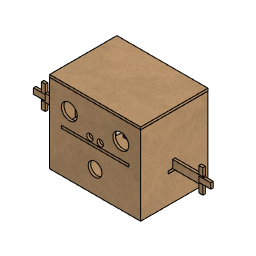
CAD finished (Autodesk Fusion 360 design; units mm, degrees)
Autodesk Fusion 360 part; units mm, degrees
sketch "Sketch1" plane through (0, 0, 0) normal (0, 0, 1) x (1, 0, 0)
  line L0 (-32.379468, 47.484339) -> (40, 47.484339)
  line L1 (40, 47.484339) -> (40, -5)
  line L2 (40, -5) -> (-32.379468, -5)
  line L3 (-32.379468, -5) -> (-32.379468, 47.484339)
  constraint horizontal L0
  constraint vertical L1
  constraint horizontal L2
  constraint vertical L3
sketch "Sketch2" plane through (0, 0, 0) normal (0, 0, 1) x (1, 0, 0)
sketch "Sketch3" plane through (0, 0, 0) normal (0, 0, 1) x (1, 0, 0)
  line L0 (-70, 30) -> (-16.7, 30)
  line L1 (-16.7, 30) -> (-16.7, -38.6)
  line L2 (-16.7, -38.6) -> (-70, -38.6)
  line L3 (-70, -38.6) -> (-70, 30)
  dimension "d3" = 53.3
  dimension "d4" = 68.6
  constraint horizontal L0
  constraint vertical L1
  constraint horizontal L2
  constraint vertical L3
  measures "d3" distance of L0.start L0.end
  measures "d4" distance of L0.start L2.end
extrude "Extrude2" add sketch "Sketch3" along normal blind 10 contours L0 L1 L2 L3 picked at (-34.466667, -15.733333) makes body 1
move_body "Move3" bodies 1 to x (0, -1, 0) y (1, 0, 0) z (0, 0, 1) at (-31.4, -108.6, 0)
move_body "Move4" bodies 1 to x (1, 0, 0) y (0, 1, 0) z (0, 0, 1) at (-5.934669, 58.827333, -1.64215)
sketch "Sketch4" plane through (0, 0, 0) normal (0, 0, 1) x (1, 0, 0)
  line L0 (40, 25) -> (125, 25)
  line L1 (125, 25) -> (125, -30)
  line L2 (125, -30) -> (40, -30)
  line L3 (40, -30) -> (40, 25)
  dimension "d7" = 85
  dimension "d8" = 55
  constraint horizontal L0
  constraint vertical L1
  constraint horizontal L2
  constraint vertical L3
  measures "d7" distance of L0.start L0.end
  measures "d8" distance of L0.start L2.end
extrude "Extrude3" add sketch "Sketch4" along normal blind 10 separate body contours L0 L1 L2 L3 picked at (68.333333, 6.666667) makes body 2
move_body "Move5" bodies 1 to x (0, 1, 0) y (-1, 0, 0) z (0, 0, 1) at (-109.007335, 42.862002, 0)
move_body "Move6" bodies 1 to x (1, 0, 0) y (0, 1, 0) z (0, 0, 1) at (69.290138, 3.072667, 11.64215)
move_body "Move7" bodies 2 to x (0, 1, 0) y (-1, 0, 0) z (0, 0, 1) at (10, -70, 0)
move_body "Move8" bodies 2 to x (1, 0, 0) y (0, 1, 0) z (0, 0, 1) at (13.481554, 0.965731, 8.735429)
sketch "Sketch5" plane through (0, 0, 0) normal (0, 0, 1) x (1, 0, 0)
  line L0 (100, -150) -> (-130, -150)
  line L1 (-130, -150) -> (-130, 20)
  line L2 (-130, 20) -> (100, 20)
  line L3 (100, 20) -> (100, -150)
  dimension "d11" = 230
  dimension "d12" = 170
  constraint horizontal L0
  constraint vertical L1
  constraint horizontal L2
  constraint vertical L3
  measures "d11" distance of L0.start L0.end
  measures "d12" distance of L0.start L2.end
extrude "Extrude4" add sketch "Sketch5" against normal blind 200 separate body contours L0 L1 L2 L3 picked at (-53.333333, -93.333333) makes body 3
sketch "Sketch6" plane through (0, 0, -200) normal (0, 0, -1) x (1, 0, 0)
  line L0 (-130, -20) -> (100, -20)
  line L1 (100, -20) -> (100, 150)
  line L2 (100, 150) -> (-130, 150)
  line L3 (-130, 150) -> (-130, -20)
  line L4 (-122.888911, 140.96297) -> (94.411089, 140.96297)
  line L5 (94.411089, 140.96297) -> (94.411089, -12.73703)
  line L6 (94.411089, -12.73703) -> (-122.888911, -12.73703)
  line L7 (-122.888911, -12.73703) -> (-122.888911, 140.96297)
  dimension "d15" = 217.3
  dimension "d16" = 153.7
  constraint horizontal L4
  constraint vertical L5
  constraint horizontal L6
  constraint vertical L7
extrude "Extrude5" cut sketch "Sketch6" against normal blind 193.35 contours L4 L5 L6 L7 picked at (-50.455578, 89.729637) bodies 3
move_body "Move9" bodies 1 to x (1, 0, 0) y (0, 1, 0) z (0, 0, 1) at (-192.155267, -38.643573, -133.723853)
move_body "Move10" bodies 2 to x (1, 0, 0) y (0, 1, 0) z (0, 0, 1) at (-190.142564, -42.930176, -139.080704)
sketch "Sketch7" plane through (0, 0, 0) normal (0, 0, 1) x (1, 0, 0)
  line L0 (-116.722098, 87.554715) -> (113.277902, 87.554715)
  line L1 (113.277902, 87.554715) -> (113.277902, 257.554715)
  line L2 (113.277902, 257.554715) -> (-116.722098, 257.554715)
  line L3 (-116.722098, 257.554715) -> (-116.722098, 87.554715)
  dimension "d19" = 230
  dimension "d20" = 170
  constraint horizontal L0
  constraint vertical L1
  constraint horizontal L2
  constraint vertical L3
extrude "Extrude6" add sketch "Sketch7" along normal blind 6.35 separate body contours L0 L1 L2 L3 picked at (-40.055431, 200.888048) makes body 4
move_body "Move11" bodies 4 to x (1, 0, 0) y (0, 1, 0) z (0, 0, 1) at (-13.20842, -237.892283, -206.176126)
sketch "Sketch8" plane through (0, 20, 0) normal (0, 1, 0) x (-1, 0, 0)
  line L0 (130, 0) -> (-100, 0)
  line L1 (-100, 0) -> (-100, -200)
  line L2 (-100, -200) -> (130, -200)
  line L3 (130, -200) -> (130, 0)
  line L4 (100, -110) -> (-72.739623, -110)
  line L5 (-72.739623, -110) -> (-72.739623, -103.65)
  line L6 (-72.739623, -103.65) -> (100, -103.65)
  line L7 (100, -103.65) -> (100, -110)
  dimension "d23" = 6.35
  constraint horizontal L4
  constraint vertical L5
  constraint horizontal L6
  constraint vertical L7
  measures "d23" distance of L4.start L6.end
extrude "Extrude7" cut sketch "Sketch8" against normal blind 200 contours L4 L5 L6 L7 picked at (42.420126, -107.883333) bodies 3
sketch "Sketch9" plane through (0, 0, 0) normal (0, 0, 1) x (1, 0, 0)
  line L0 (-120, 110) -> (52.74, 110)
  line L1 (52.74, 110) -> (52.74, 280)
  line L2 (52.74, 280) -> (-120, 280)
  line L3 (-120, 280) -> (-120, 110)
  dimension "d26" = 172.74
  dimension "d27" = 170
  constraint horizontal L0
  constraint vertical L1
  constraint horizontal L2
  constraint vertical L3
  measures "d26" distance of L0.start L0.end
  measures "d27" distance of L0.start L2.end
extrude "Extrude8" add sketch "Sketch9" against normal blind 6.35 separate body contours L0 L1 L2 L3 picked at (-62.42, 166.666667) makes body 5
move_body "Move12" bodies 5 to x (1, 0, 0) y (0, 1, 0) z (0, 0, 1) at (20.106965, -259.503239, -103.236774)
sketch "Sketch10" plane through (0, -150, 0) normal (0, -1, 0) x (1, 0, 0)
  line L0 (72.739623, -103.65) -> (72.739623, -110)
  line L1 (72.739623, -110) -> (-100, -110)
  line L2 (-100, -110) -> (-100, -103.65)
  line L3 (-100, -103.65) -> (72.739623, -103.65)
  line L4 (100, 0) -> (-130, 0)
  line L5 (-130, 0) -> (-130, -200)
  line L6 (-130, -200) -> (100, -200)
  line L7 (100, -200) -> (100, 0)
  circle A0 centre (50, -150) radius 20
  circle A1 centre (50, -150) radius 20
  circle A2 centre (-80, -150) radius 20
extrude "Extrude9" cut sketch "Sketch10" against normal blind 20 contours A0 A1 | A2 picked at (55.729979, -143.285883) picked at (-74.270021, -143.285883) bodies 3
sketch "Sketch11" plane through (0, -150, 0) normal (0, -1, 0) x (1, 0, 0)
  circle A0 centre (-80, -150) radius 20
  circle A1 centre (50, -150) radius 20
  line L0 (72.739623, -103.65) -> (72.739623, -110)
  line L1 (72.739623, -110) -> (-100, -110)
  line L2 (-100, -110) -> (-100, -103.65)
  line L3 (-100, -103.65) -> (72.739623, -103.65)
  line L4 (100, 0) -> (-130, 0)
  line L5 (-130, 0) -> (-130, -200)
  line L6 (-130, -200) -> (100, -200)
  line L7 (100, -200) -> (100, 0)
  circle A2 centre (-1.949729, -120.049809) radius 8.05
  dimension "d32" = 16.1
  measures "d32" diameter of A2
sketch "Sketch12" plane through (0, -150, 0) normal (0, -1, 0) x (1, 0, 0)
sketch "Sketch13" plane through (0, -150, 0) normal (0, -1, 0) x (1, 0, 0)
  circle A0 centre (-28.05, -120.05) radius 8.05
  dimension "d33" = 16.1
  measures "d33" diameter of A0
extrude "Extrude10" cut sketch "Sketch11" sketch "Sketch13" against normal blind 10 contours A2 picked at (-2.546826, -117.670176) of sketch 2 contours A0 picked at (-28.647098, -117.433943) bodies 3
move_body "Move13" bodies 4 to x (1, 0, 0) y (0, 1, 0) z (0, 0, 1) at (231.754055, -19.247754, 6.176126)
move_body "Move14" bodies 2 to x (1, 0, 0) y (0, 1, 0) z (0, 0, 1) at (189.899012, -32.028626, 10.567885)
move_body "Move15" bodies 1 to x (1, 0, 0) y (0, 1, 0) z (0, 0, 1) at (183.687801, -30.675834, -12.288573)
move_body "Move16" bodies 1 to x (1, 0, 0) y (0, 1, 0) z (0, 0, 1) at (0, 0, 15)
sketch "Sketch14" plane through (100, 0, 0) normal (1, 0, 0) x (0, 1, 0)
sketch "Sketch15" plane through (100, 0, 0) normal (1, 0, 0) x (0, 1, 0)
  line L0 (-50, -75) -> (-80, -75)
  line L1 (-80, -75) -> (-80, -68.65)
  line L2 (-80, -68.65) -> (-50, -68.65)
  line L3 (-50, -68.65) -> (-50, -75)
  dimension "d36" = 6.35
  constraint horizontal L0
  constraint vertical L1
  constraint horizontal L2
  constraint vertical L3
  measures "d36" distance of L0.start L2.end
extrude "Extrude11" cut sketch "Sketch15" against normal blind 320 contours L0 L1 L2 L3 picked at (-70, -72.883333) bodies 3
sketch "Sketch16" plane through (0, 0, 0) normal (0, 0, 1) x (1, 0, 0)
  line L0 (-100, 140) -> (130, 140)
  line L1 (130, 140) -> (130, 170)
  line L2 (130, 170) -> (-100, 170)
  line L3 (-100, 170) -> (-100, 140)
  dimension "d39" = 230
  dimension "d40" = 30
  constraint horizontal L0
  constraint vertical L1
  constraint horizontal L2
  constraint vertical L3
  measures "d39" distance of L0.start L0.end
  measures "d40" distance of L0.start L2.end
extrude "Extrude12" add sketch "Sketch16" against normal blind 6.35 separate body contours L0 L1 L2 L3 picked at (-23.333333, 150) makes body 6
move_body "Move17" bodies 6 to x (1, 0, 0) y (0, 1, 0) z (0, 0, 1) at (-29.739923, -217.865341, -68.375414)
move_body "Move18" bodies 6 to x (1, 0, 0) y (0, 1, 0) z (0, 0, 1) at (0, -2.152, 0)
sketch "Sketch17" plane through (0, 0, -74.725414) normal (0, 0, -1) x (1, 0, 0)
  line L0 (-129.739923, 80.017341) -> (-129.739923, 50.017341)
  line L1 (-129.739923, 50.017341) -> (100.260077, 50.017341)
  line L2 (100.260077, 50.017341) -> (100.260077, 80.017341)
  line L3 (100.260077, 80.017341) -> (-129.739923, 80.017341)
sketch "Sketch18" plane through (0, 0, -74.725414) normal (0, 0, -1) x (1, 0, 0)
  line L0 (90.260001, 76.717001) -> (86.610001, 76.717001)
  line L1 (86.610001, 76.717001) -> (86.610001, 64.717001)
  line L2 (86.610001, 64.717001) -> (90.260001, 64.717001)
  line L3 (90.260001, 64.717001) -> (90.260001, 76.717001)
  dimension "d43" = 3.65
  constraint horizontal L0
  constraint vertical L1
  constraint horizontal L2
  constraint vertical L3
sketch "Sketch19" plane through (0, 0, -74.725414) normal (0, 0, -1) x (1, 0, 0)
  line L0 (60.610001, 64.717001) -> (56.960001, 64.717001)
  line L1 (56.960001, 64.717001) -> (56.960001, 76.717001)
  line L2 (56.960001, 76.717001) -> (60.610001, 76.717001)
  line L3 (60.610001, 76.717001) -> (60.610001, 64.717001)
  dimension "d44" = 3.65
  constraint horizontal L0
  constraint vertical L1
  constraint horizontal L2
  constraint vertical L3
extrude "Extrude13" cut sketch "Sketch18" against normal blind 11 contours L0 L1 L2 L3 picked at (87.826668, 72.717001) bodies 6
extrude "Extrude14" cut sketch "Sketch19" against normal blind 22 contours L0 L1 L2 L3 picked at (58.176668, 68.717001) bodies 6
sketch "Sketch20" plane through (0, 0, 0) normal (0, 0, 1) x (1, 0, 0)
  line L0 (95, -105) -> (91.35, -105)
  line L1 (91.35, -105) -> (91.35, -117)
  line L2 (91.35, -117) -> (95, -117)
  line L3 (95, -117) -> (95, -105)
  dimension "d49" = 3.65
  dimension "d50" = 12
  constraint horizontal L0
  constraint vertical L1
  constraint horizontal L2
  constraint vertical L3
  measures "d49" distance of L0.start L0.end
  measures "d50" distance of L0.start L2.end
sketch "Sketch21" plane through (0, 0, 0) normal (0, 0, 1) x (1, 0, 0)
  line L0 (65.35, -105) -> (61.7, -105)
  line L1 (61.7, -105) -> (61.7, -117)
  line L2 (61.7, -117) -> (65.35, -117)
  line L3 (65.35, -117) -> (65.35, -105)
  dimension "d51" = 3.65
  dimension "d52" = 12
  constraint horizontal L0
  constraint vertical L1
  constraint horizontal L2
  constraint vertical L3
  measures "d51" distance of L0.start L0.end
  measures "d52" distance of L0.start L2.end
extrude "Extrude15" add sketch "Sketch21" against normal blind 25 separate body contours L0 L1 L2 L3 picked at (62.916667, -109) makes body 7
extrude "Extrude16" add sketch "Sketch20" against normal blind 25 separate body contours L0 L1 L2 L3 picked at (92.566667, -109) makes body 8
extrude "Extrude17" cut 1 faces at (86.610001, -72.717001, -72.608747) along direction (-1, 0, 0) blind 2.65 on bodies 6 bodies 6
extrude "Extrude18" cut 1 faces at (83.960001, -72.717001, -72.608747) along direction (-1, 0, 0) blind 0.05 on bodies 6 bodies 6
extrude "Extrude19" cut 1 faces at (56.960001, -68.717001, -72.608747) along direction (-1, 0, 0) blind 6.35 on bodies 6 bodies 6
extrude "Extrude20" add 1 faces at (60.610001, -72.717001, -72.608747) along direction (-1, 0, 0) blind 3.3 on bodies 6 bodies 6
extrude "Extrude21" cut 1 faces at (57.310001, -72.717001, -72.608747) along direction (1, 0, 0) blind 0.6 on bodies 6 bodies 6
extrude "Extrude22" add 1 faces at (50.610001, -68.717001, -72.608747) along direction (1, 0, 0) blind 0.95 on bodies 6 bodies 6
extrude "Extrude23" add 1 faces at (91.35, -109, -8.333333) along direction (-1, 0, 0) blind 0.7 on bodies 8 bodies 8
extrude "Extrude24" cut 1 faces at (65.35, -113, -8.333333) along direction (-1, 0, 0) blind 0.7 on bodies 7 bodies 7
extrude "Extrude25" add 1 faces at (61.7, -109, -8.333333) along direction (-1, 0, 0) blind 1.4 on bodies 7 bodies 7
extrude "Extrude26" add 1 faces at (90.65, -109, -8.333333) along direction (-1, 0, 0) blind 2 on bodies 8 bodies 8
extrude "Extrude27" cut 1 faces at (64.65, -113, -8.333333) along direction (-1, 0, 0) blind 2 on bodies 7 bodies 7
extrude "Extrude28" add 1 faces at (60.3, -109, -8.333333) along direction (-1, 0, 0) blind 4 on bodies 7 bodies 7
sketch "Sketch22" plane through (56.3, 0, 0) normal (-1, 0, 0) x (0, -1, 0)
extrude "Extrude29" cut 1 faces at (86.026668, -64.717001, -70.492081) along direction (0, 1, 0) blind 10 on bodies 6 bodies 6
extrude "Extrude30" cut 1 faces at (53.676668, -64.717001, -70.492081) along direction (0, 1, 0) blind 10 on bodies 6 bodies 6
extrude "Extrude31" add 1 faces at (60.533333, -105, -8.333333) along direction (0, 1, 0) blind 10 on bodies 7 bodies 7
extrude "Extrude32" add 1 faces at (92.883333, -105, -8.333333) along direction (0, 1, 0) blind 10 on bodies 8 bodies 8
sketch "Sketch23" plane through (56.3, 0, 0) normal (-1, 0, 0) x (0, -1, 0)
  line L0 (113.499806, -12.749811) -> (98.499806, -12.749811)
  line L1 (98.499806, -12.749811) -> (98.499806, -6.399811)
  line L2 (98.499806, -6.399811) -> (113.499806, -6.399811)
  line L3 (113.499806, -6.399811) -> (113.499806, -12.749811)
  dimension "d91" = 15
  dimension "d92" = 6.35
  constraint horizontal L0
  constraint vertical L1
  constraint horizontal L2
  constraint vertical L3
extrude "Extrude33" add 1 faces at (60.533333, -109.666667, -25) along direction (0, 0, -1) blind 5.85 on bodies 7 bodies 7
extrude "Extrude34" add 1 faces at (90.766667, -102.333333, -25) along direction (0, 0, -1) blind 5.85 on bodies 8 bodies 8
sketch "Sketch24" plane through (56.3, 0, 0) normal (-1, 0, 0) x (0, -1, 0)
  line L0 (95, -30.85) -> (117, -30.85)
  line L1 (113.500002, -31) -> (98.500002, -31)
  line L2 (98.500002, -31) -> (98.500002, -24.65)
  line L3 (98.500002, -24.65) -> (113.500002, -24.65)
  line L4 (113.500002, -24.65) -> (113.500002, -31)
  dimension "d97" = 15
  dimension "d98" = 6.35
  constraint horizontal L1
  constraint vertical L2
  constraint horizontal L3
  constraint vertical L4
extrude "Extrude35" add 1 faces at (60.533333, -109.666667, -30.85) along direction (0, 0, -1) blind 3 on bodies 7 bodies 7
extrude "Extrude36" add 1 faces at (90.766667, -102.333333, -30.85) along direction (0, 0, -1) blind 3 on bodies 8 bodies 8
extrude "Extrude37" cut sketch "Sketch24" against normal blind 41 contours L0 L2 L3 L4 picked at (103.500002, -28.783333) bodies 7 8
extrude "Extrude38" cut sketch "Sketch23" against normal blind 39 contours L0 L1 L2 L3 picked at (103.499806, -10.633144) bodies 7 8
sketch "Sketch25" plane through (0, 0, 0) normal (0, 0, 1) x (1, 0, 0)
  line L0 (55.000001, -135.000002) -> (93.700001, -135.000002)
  line L1 (93.700001, -135.000002) -> (93.700001, -150.000002)
  line L2 (93.700001, -150.000002) -> (55.000001, -150.000002)
  line L3 (55.000001, -150.000002) -> (55.000001, -135.000002)
  dimension "d107" = 38.7
  constraint horizontal L0
  constraint vertical L1
  constraint horizontal L2
  constraint vertical L3
extrude "Extrude39" add sketch "Sketch25" along normal blind 6.35 separate body contours L0 L1 L2 L3 picked at (67.900001, -140.000002) makes body 9
move_body "Move19" bodies 9 to x (1, 0, 0) y (0, 1, 0) z (0, 0, 1) at (1.303223, 36.558885, -12.752949)
sketch "Sketch26" plane through (0, 0, 0) normal (0, 0, 1) x (1, 0, 0)
  line L0 (-30, 12) -> (8.7, 12)
  line L1 (8.7, 12) -> (8.7, -3)
  line L2 (8.7, -3) -> (-30, -3)
  line L3 (-30, -3) -> (-30, 12)
  dimension "d110" = 38.7
  dimension "d111" = 15
  constraint horizontal L0
  constraint vertical L1
  constraint horizontal L2
  constraint vertical L3
  measures "d110" distance of L0.start L0.end
  measures "d111" distance of L0.start L2.end
extrude "Extrude40" add sketch "Sketch26" along normal blind 6.35 separate body contours L0 L1 L2 L3 picked at (-17.1, 7) makes body 10
move_body "Move20" bodies 10 to x (1, 0, 0) y (0, 1, 0) z (0, 0, 1) at (86.347136, -110.477197, -31.06443)
move_body "Move21" bodies 7 8 9 10 to x (1, 0, 0) y (0, 1, 0) z (0, 0, 1) at (-4.838405, 40.47214, -68.412026)
move_body "Move22" bodies 4 to x (1, 0, 0) y (0, 1, 0) z (0, 0, 1) at (-231.998044, 19.570387, 0)
sketch "Sketch27" plane through (94.411089, 0, 0) normal (-1, 0, 0) x (0, -1, 0)
  line L0 (80, -68.65) -> (80, -75)
  line L1 (80, -75) -> (50, -75)
  line L2 (50, -75) -> (50, -68.65)
  line L3 (50, -68.65) -> (80, -68.65)
  line L4 (-12.73703, -200) -> (140.96297, -200)
  line L5 (140.96297, -200) -> (140.96297, -6.65)
  line L6 (140.96297, -6.65) -> (-12.73703, -6.65)
  line L7 (-12.73703, -6.65) -> (-12.73703, -200)
  line L8 (95, -75) -> (88.65, -75)
  line L9 (88.65, -75) -> (88.65, -111.76823)
  line L10 (88.65, -111.76823) -> (95, -111.76823)
  line L11 (95, -111.76823) -> (95, -75)
  dimension "d114" = 6.35
  constraint horizontal L8
  constraint vertical L9
  constraint horizontal L10
  constraint vertical L11
  measures "d114" distance of L8.start L8.end
extrude "Extrude41" add 1 faces at (72.739623, -143.975314, -107.883333) along direction (-1, 0, 0) blind 2.74 on bodies 3 bodies 3
extrude "Extrude42" cut 1 faces at (72.846965, -92.836573, -105.35344) along direction (-1, 0, 0) blind 2.74 on bodies 5 bodies 5
move_body "Move23" bodies 5 to x (1, 0, 0) y (0, 1, 0) z (0, 0, 1) at (0.184253, 0, -0.368506)
extrude "Extrude43" add 1 faces at (72.739623, 17.57901, -107.883333) along direction (-1, 0, 0) blind 2.74 on bodies 3 bodies 3
extrude "Extrude44" cut sketch "Sketch27" against normal blind 15 contours L8 L9 L10 L11 picked at (90.766667, -87.256077) bodies 3
extrude "Extrude45" cut 1 faces at (98.13703, -90.766667, -111.76823) along direction (0, 0, -1) blind 28 on bodies 3 bodies 3
extrude "Extrude46" cut 1 faces at (96.274059, -95, -118.17882) along direction (0, -1, 0) blind 1.5 on bodies 3 bodies 3
sketch "Sketch28" plane through (0, 0, 0) normal (0, 0, 1) x (1, 0, 0)
  line L0 (60, 60) -> (180, 60)
  line L1 (180, 60) -> (180, 80)
  line L2 (180, 80) -> (60, 80)
  line L3 (60, 80) -> (60, 60)
  constraint horizontal L0
  constraint vertical L1
  constraint horizontal L2
  constraint vertical L3
extrude "Extrude47" add sketch "Sketch28" along normal blind 6.35 separate body contours L0 L1 L2 L3 picked at (100, 73.333333) makes body 11
extrude "Extrude48" add 1 faces at (94.411089, -8.175314, -93.883333) along direction (-1, 0, 0) blind 0.761 on bodies 3 bodies 3 7 8 9 10 6
extrude "Extrude49" cut 1 faces at (13.586933, -140.96297, -38.983333) along direction (0, -1, 0) blind 2.687 on bodies 3 bodies 3
extrude "Extrude50" cut 1 faces at (-122.888911, -70.304314, -158.333333) along direction (-1, 0, 0) blind 0.761 on bodies 3 bodies 3
extrude "Extrude51" cut 1 faces at (13.333267, 12.73703, -38.983333) along direction (0, 1, 0) blind 0.913 on bodies 3 bodies 3
sketch "Sketch29" plane through (0, 0, 0) normal (0, 0, 1) x (1, 0, 0)
  line L0 (175, 45) -> (205, 45)
  line L1 (205, 45) -> (205, 55)
  line L2 (205, 55) -> (175, 55)
  line L3 (175, 55) -> (175, 45)
  dimension "d139" = 30
  dimension "d140" = 10
  constraint horizontal L0
  constraint vertical L1
  constraint horizontal L2
  constraint vertical L3
  measures "d139" distance of L0.start L0.end
  measures "d140" distance of L0.start L2.end
extrude "Extrude52" add sketch "Sketch29" along normal blind 6.35 separate body contours L0 L1 L2 L3 picked at (185, 51.666667) makes body 12
move_body "Move24" bodies 12 to x (0.64278761, -0.76604444, 0) y (0.76604444, 0.64278761, 0) z (0, 0, 1) at (20.332568, 165.021548, 1.313402)
move_body "Move25" bodies 12 to x (1, 0, 0) y (0, 1, 0) z (0, 0, 1) at (0, 0, -1)
move_body "Move26" bodies 12 to x (1, 0, 0) y (0, 1, 0) z (0, 0, 1) at (0, 0, -0.31)
move_body "Move27" bodies 12 to x (0.76604444, -0.64278761, 0) y (0.64278761, 0.76604444, 0) z (0, 0, 1) at (15.415059, 116.168285, 0)
move_body "Move28" bodies 12 to x (1, 0, 0) y (0, 1, 0) z (0, 0, 1) at (-12, 7, 0)
move_body "Move29" bodies 12 to x (1, 0, 0) y (0, 1, 0) z (0, 0, 1) at (-0.065, 0, 0)
move_body "Move30" bodies 12 to x (1, 0, 0) y (0, 1, 0) z (0, 0, 1) at (0, 8.487, 0)
sketch "Sketch30" plane through (0, 0, 0) normal (0, 0, 1) x (1, 0, 0)
  line L0 (158.55408, 93.327582) -> (188.55408, 93.327582)
  line L1 (188.55408, 93.327582) -> (188.55408, 103.327582)
  line L2 (188.55408, 103.327582) -> (158.55408, 103.327582)
  line L3 (158.55408, 103.327582) -> (158.55408, 93.327582)
  dimension "d143" = 30
  dimension "d144" = 10
  constraint horizontal L0
  constraint vertical L1
  constraint horizontal L2
  constraint vertical L3
extrude "Extrude53" add sketch "Sketch30" along normal blind 6.35 separate body contours L0 L1 L2 L3 picked at (168.55408, 99.994248) makes body 13
move_body "Move31" bodies 13 to x (0, 1, 0) y (-1, 0, 0) z (0, 0, 1) at (272.881662, -79.226498, 0)
move_body "Move32" bodies 13 to x (1, 0, 0) y (0, 1, 0) z (0, 0, 1) at (0.446, 0, 0)
move_body "Move33" bodies 13 to x (1, 0, 0) y (0, 1, 0) z (0, 0, 1) at (0, -9.328, 0)
sketch "Sketch31" plane through (0, 0, 0) normal (0, 0, 1) x (1, 0, 0)
  line L0 (185, 65) -> (215, 65)
  line L1 (215, 65) -> (215, 75)
  line L2 (215, 75) -> (185, 75)
  line L3 (185, 75) -> (185, 65)
  dimension "d147" = 30
  dimension "d148" = 10
  constraint horizontal L0
  constraint vertical L1
  constraint horizontal L2
  constraint vertical L3
  measures "d147" distance of L0.start L0.end
  measures "d148" distance of L0.start L2.end
extrude "Extrude54" add sketch "Sketch31" along normal blind 6.35 separate body contours L0 L1 L2 L3 picked at (195, 71.666667) makes body 14
move_body "Move34" bodies 14 to x (1, 0, 0) y (0, 1, 0) z (0, 0, 1) at (-12.505099, 0.002416, -0.034416)
move_face "MoveFace1" by (0, 0.002, 0) 1 faces at (182.494901, 71.669083, -0.034416) on bodies 14
move_body "Move35" bodies 14 to x (1, 0, 0) y (0, 1, 0) z (0, 0, 1) at (0, 0.002, 0)
move_body "Move36" bodies 14 to x (1, 0, 0) y (0, 1, 0) z (0, 0, 1) at (-2.495, 0, 0)
move_body "Move37" bodies 11 14 12 13 to x (1, 0, 0) y (0, 0, -1) z (0, 1, 0) at (0, -95.739602, -20.36563)
extrude "Extrude55" add 1 faces at (179.999901, -93.657351, -85.370046) along direction (0, 0, 1) blind 2 on bodies 14 bodies 14 13 11 12
extrude "Extrude56" add 1 faces at (193.333268, -93.645879, -95.370046) along direction (0, 0, -1) blind 2 on bodies 14 bodies 14 13
extrude "Extrude57" cut 1 faces at (95.766726, -88.65, -118.17882) along direction (0, 1, 0) blind 5 on bodies 3 bodies 3
move_body "Move38" bodies 14 to x (1, 0, 0) y (0, 1, 0) z (0, 0, 1) at (0, 5, 0)
extrude "Extrude58" add 1 faces at (97.883363, -96.5, -118.17882) along direction (0, 1, 0) blind 5 on bodies 3 bodies 3
move_body "Move39" bodies 1 to x (1, 0, 0) y (0, 1, 0) z (0, 0, 1) at (-20, 0, 0)
move_body "Move40" bodies 2 to x (1, 0, 0) y (0, 1, 0) z (0, 0, 1) at (-20, 0, 0)
sketch "Sketch32" plane through (0, 0, -109.95528) normal (0, 0, -1) x (1, 0, 0)
  line L0 (70.291218, -20.496761) -> (70.291218, 149.503239)
  line L1 (70.291218, 149.503239) -> (-99.708782, 149.503239)
  line L2 (-99.708782, 149.503239) -> (-99.708782, -20.496761)
  line L3 (-99.708782, -20.496761) -> (70.291218, -20.496761)
  line L4 (70.291218, 83.901333) -> (45.165554, 83.901333)
  line L5 (45.165554, 83.901333) -> (45.165554, 90.361333)
  line L6 (45.165554, 90.361333) -> (70.291218, 90.361333)
  line L7 (70.291218, 90.361333) -> (70.291218, 83.901333)
  dimension "d159" = 6.46
  constraint horizontal L4
  constraint vertical L5
  constraint horizontal L6
  constraint vertical L7
extrude "Extrude59" cut sketch "Sketch32" against normal blind 7 contours L0 L4 L5 L6 L7 picked at (61.915997, 86.054666) bodies 5
extrude "Extrude60" cut 1 faces at (53.540775, -90.361333, -107.838613) along direction (0, -1, 0) blind 1 on bodies 5 bodies 5
sketch "Sketch33" plane through (0, -150, 0) normal (0, -1, 0) x (1, 0, 0)
  circle A0 centre (-1.949729, -120.049809) radius 8.05
  circle A1 centre (-28.05, -120.05) radius 8.05
  circle A2 centre (-80, -150) radius 20
  circle A3 centre (50, -150) radius 20
  line L0 (69.999623, -103.65) -> (69.999623, -110)
  line L1 (69.999623, -110) -> (-100, -110)
  line L2 (-100, -110) -> (-100, -103.65)
  line L3 (-100, -103.65) -> (69.999623, -103.65)
  line L4 (100, 0) -> (-130, 0)
  line L5 (-130, 0) -> (-130, -200)
  line L6 (-130, -200) -> (100, -200)
  line L7 (100, -200) -> (100, 0)
  circle A4 centre (-15.000189, -56.149806) radius 17.5
  dimension "d164" = 35
  measures "d164" diameter of A4
extrude "Extrude61" cut sketch "Sketch33" against normal blind 15 contours A4 picked at (-9.685173, -56.149806) bodies 3
copy_body "CopyPasteBodies1" bodies 14 makes body 15
move_body "Move41" bodies 15 to x (-1, 0, 0) y (0, 1, 0) z (0, 0, -1) at (-145.610071, 24.696765, -200.232505)
combine "Combine1" operation add target body 7 tool bodies 8 10 9
sketch "Sketch34" plane through (0, 0, -74.725414) normal (0, 0, -1) x (1, 0, 0)
  line L0 (90.260001, 76.717001) -> (90.260001, 54.717001)
  line L1 (90.260001, 54.717001) -> (83.910001, 54.717001)
  line L2 (83.910001, 54.717001) -> (83.910001, 76.717001)
  line L3 (83.910001, 76.717001) -> (90.260001, 76.717001)
  line L4 (100, 80.017341) -> (100, 80)
  line L5 (100, 80) -> (93.650089, 80)
  line L6 (93.650089, 80) -> (93.650089, 80.017341)
  line L7 (93.650089, 80.017341) -> (-123.649911, 80.017341)
  line L8 (-123.649911, 80.017341) -> (-123.649911, 80)
  line L9 (-123.649911, 80) -> (-129.739923, 80)
  line L10 (-129.739923, 80) -> (-129.739923, 50.017341)
  line L11 (-129.739923, 50.017341) -> (100.260077, 50.017341)
  line L12 (100.260077, 50.017341) -> (100.260077, 80.017341)
  line L13 (100.260077, 80.017341) -> (100, 80.017341)
  line L14 (51.560001, 54.717001) -> (51.560001, 76.717001)
  line L15 (51.560001, 76.717001) -> (57.910001, 76.717001)
  line L16 (57.910001, 76.717001) -> (57.910001, 54.717001)
  line L17 (57.910001, 54.717001) -> (51.560001, 54.717001)
  line L18 (-118.199245, 75.684647) -> (-111.849245, 75.684647)
  line L19 (-111.849245, 75.684647) -> (-111.849245, 53.684647)
  line L20 (-111.849245, 53.684647) -> (-118.199245, 53.684647)
  line L21 (-118.199245, 53.684647) -> (-118.199245, 75.684647)
  line L22 (-85.849646, 54.619041) -> (-85.849646, 76.619041)
  line L23 (-85.849646, 76.619041) -> (-79.499646, 76.619041)
  line L24 (-79.499646, 76.619041) -> (-79.499646, 54.619041)
  line L25 (-79.499646, 54.619041) -> (-85.849646, 54.619041)
  dimension "d167" = 6.35
  dimension "d168" = 22
  dimension "d169" = 6.35
  dimension "d170" = 22
  constraint horizontal L18
  constraint vertical L19
  constraint horizontal L20
  constraint vertical L21
  constraint horizontal L23
  constraint vertical L24
  constraint horizontal L25
  constraint vertical L22
extrude "Extrude62" cut sketch "Sketch34" against normal blind 9 contours L18 L19 L20 L21 | L22 L23 L24 L25 picked at (-116.082578, 68.351314) picked at (-83.73298, 61.952375) bodies 3
sketch "Sketch35" plane through (0, 0, 0) normal (0, 0, 1) x (1, 0, 0)
  line L0 (-140, 50) -> (-133.65, 50)
  line L1 (-133.65, 50) -> (-133.65, 72)
  line L2 (-133.65, 72) -> (-140, 72)
  line L3 (-140, 72) -> (-140, 50)
  line L4 (-107.65, 72) -> (-107.65, 50)
  line L5 (-107.65, 50) -> (-101.3, 50)
  line L6 (-101.3, 50) -> (-101.3, 72)
  line L7 (-101.3, 72) -> (-107.65, 72)
  dimension "d173" = 6.35
  dimension "d174" = 22
  dimension "d175" = 6.35
  dimension "d176" = 22
  constraint horizontal L0
  constraint vertical L1
  constraint horizontal L2
  constraint vertical L3
  constraint horizontal L5
  constraint vertical L6
  constraint horizontal L7
  constraint vertical L4
  measures "d173" distance of L0.start L0.end
  measures "d174" distance of L0.start L2.end
  measures "d175" distance of L4.end L5.end
  measures "d176" distance of L4.end L4.start
extrude "Extrude63" add sketch "Sketch35" against normal blind 25 separate body contours L0 L1 L2 L3 | L4 L5 L6 L7 picked at (-137.883333, 64.666667) picked at (-105.533333, 64.666667) makes body 16 at (-140, 64.666667, -8.333333) makes body 17 at (-101.3, 57.333333, -8.333333)
extrude "Extrude64" add 2 faces at (-105.533333, 64.666667, -25) (-137.883333, 64.666667, -25) along direction (0, 0, -1) blind 8.85 on bodies 16 17 bodies 17 16
sketch "Sketch36" plane through (-101.3, 0, 0) normal (1, 0, 0) x (0, 1, 0)
  line L0 (72, 0) -> (50, 0)
  line L1 (50, 0) -> (50, -33.85)
  line L2 (50, -33.85) -> (72, -33.85)
  line L3 (72, -33.85) -> (72, 0)
  line L4 (64.180001, -29) -> (57.820001, -29)
  line L5 (57.820001, -29) -> (57.820001, -9)
  line L6 (57.820001, -9) -> (64.180001, -9)
  line L7 (64.180001, -9) -> (64.180001, -29)
  dimension "d181" = 6.36
  dimension "d182" = 20
  constraint horizontal L4
  constraint vertical L5
  constraint horizontal L6
  constraint vertical L7
extrude "Extrude65" cut sketch "Sketch36" against normal blind 5 contours L4 L5 L6 L7 picked at (59.940001, -15.666667) bodies 17
move_body "Move42" bodies 17 16 to x (1, 0, 0) y (0, 1, 0) z (0, 0, 1) at (21.91396, -126.608609, -68.279212)
move_body "Move43" bodies 16 to x (1, 0, 0) y (0, 1, 0) z (0, 0, 1) at (0, 1, 0)
move_body "Move44" bodies 16 17 to x (1, 0, 0) y (0, 1, 0) z (0, 0, 1) at (0, 0, 2)
move_body "Move45" bodies 17 16 to x (1, 0, 0) y (0, 1, 0) z (0, 0, 1) at (0, 0, 0.565)
move_body "Move46" bodies 16 17 to x (1, 0, 0) y (0, 1, 0) z (0, 0, 1) at (0, 0, -0.6)
move_body "Move47" bodies 17 to x (1, 0, 0) y (0, 1, 0) z (0, 0, 1) at (0, 0, -20)
extrude "Extrude66" cut 1 faces at (-85.849646, -61.952375, -72.608747) along direction (-1, 0, 0) blind 15 on bodies 3 bodies 3
extrude "Extrude67" add 1 faces at (-79.499646, -69.285708, -72.608747) along direction (-1, 0, 0) blind 15 on bodies 3 bodies 3
move_body "Move48" bodies 17 to x (1, 0, 0) y (0, 1, 0) z (0, 0, 1) at (-15, 0, 0)
move_body "Move49" bodies 17 to x (1, 0, 0) y (0, 1, 0) z (0, 0, 1) at (0, 0, 20)
extrude "Extrude68" cut 1 faces at (-99.38604, -64.548608, -88.647546) along direction (-1, 0, 0) blind 33 on bodies 17 bodies 3 16 17
extrude "Extrude69" cut 3 faces at (-113.852706, -66.668608, -75.314213) (-125.766608, -66.668608, -75.314213) (-98.619373, -66.668608, -75.314213) along direction (0, 0, 1) blind 0.6 on bodies 3 16 17 bodies 3 16 17
extrude "Extrude70" add 3 faces at (-125.766608, -64.548608, -95.314213) (-113.852706, -64.548608, -95.314213) (-96.502706, -64.548608, -95.314213) along direction (0, 0, 1) blind 0.6 on bodies 3 16 17 bodies 3 16 17
move_body "Move50" bodies 15 to x (1, 0, 0) y (0, 1, 0) z (0, 0, 1) at (119.280937, -2.879728, 29.352499)
move_body "Move51" bodies 15 to x (1, 0, 0) y (0, 1, 0) z (0, 0, 1) at (0, 0, -4.202)
move_body "Move52" bodies 4 to x (1, 0, 0) y (0, 1, 0) z (0, 0, 1) at (0, 0, -6.35)
extrude "Extrude71" cut 1 faces at (61.915997, -83.901333, -107.838613) along direction (0, 1, 0) blind 0.27 on bodies 5 bodies 5
extrude "Extrude72" cut 1 faces at (53.540775, -91.361333, -107.838613) along direction (0, -1, 0) blind 0.27 on bodies 5 bodies 5
move_face "MoveFace2" by (0, -0.499, 0) 1 faces at (13.624551, 20.496761, -105.721947) on bodies 5
move_face "MoveFace3" by (-0.298, 0, 0) 1 faces at (13.624551, 19.997761, -105.721947) on bodies 5
move_face "MoveFace4" by (-0.292, 0, 0) 1 faces at (13.624551, 19.997761, -105.721947) on bodies 5
move_body "Move53" bodies 5 to x (1, 0, 0) y (0, 1, 0) z (0, 0, 1) at (-0.292, 0, 0)
move_body "Move54" bodies 5 to x (1, 0, 0) y (0, 1, 0) z (0, 0, 1) at (0, 0.045, 0)
extrude "Extrude73" add 1 faces at (-43.334115, -149.458239, -105.721947) along direction (0, -1, 0) blind 0.544 on bodies 5 bodies 5 4 7 15 16 17 3
move_body "Move55" bodies 1 2 4 5 7 15 16 17 14 to x (-1, 0, 0) y (0, 1, 0) z (0, 0, -1) at (26.776478, 79.216354, 5.57537)
copy_body "Body->Comp2" bodies 14 removing the originals makes body 18 in component "Hand_R"
component "Hand_R" placed x (1, 0, 0) y (0, 1, 0) z (0, 0, 1) at (0, 0, 0)
named bodies: "Arduino", "Breadboard", "Exterior", "Roof (part of exterior)", "Arduino stand", "Servo stand", "Servo shelf", "Hand_R", "Hand_L"
